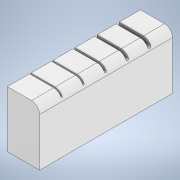
# Autodesk Inventor part: Nut0
Saved by Autodesk Inventor 2021 (Build 250183000, 183)
## iProperties
Created: 2021-02-08
Part Number: Nut0
Material: LCP Plastic
Document SubType Name: Modeling
Designer: Ryan
Density: 1.626 g/cm^3
Appearance: Smooth - White
Author: Ryan
Autodesk Inventor part; units mm, degrees
ref_plane "YZ Plane" through (0, 0, 0) normal (1, 0, 0) x (0, 1, 0)
ref_plane "XZ Plane" through (0, 0, 0) normal (0, 1, 0) x (-1, 0, 0)
ref_plane "XY Plane" through (0, 0, 0) normal (0, 0, 1) x (1, 0, 0)
sketch "Sketch1" plane through (0, 0, 0) normal (0, 1, 0) x (-1, 0, 0)
  line L0 (6.35, 26.2509) -> (-6.35, 26.2509)
  line L1 (-6.35, 26.2509) -> (-6.35, -26.2509)
  line L2 (-6.35, -26.2509) -> (6.35, -26.2509)
  line L3 (6.35, -26.2509) -> (6.35, 26.2509)
  point P0 (0, 0)
  dimension "d0" = 6.35
  dimension "d1" = 12.7
  dimension "d2" = 52.5018
  dimension "d3" = 26.2509
  constraints: 8 end point, 2 parallel, 1 horizontal, 1 perpendicular
  measures "d0" distance from line of point (0, 0) L3
  measures "d1" distance of L0.start L0.end
  measures "d2" distance of L0.end L1.end
  measures "d3" distance from line of L0 point (0, 0)
extrude "Extrusion1" add sketch "Sketch1" along normal blind 22.225
fillet "Fillet1" radius 3.175 1 edges at (6.35, 22.225, 0)
sketch "Sketch2" plane through (-6.35, 0, -26.2509) normal (-1, 0, 0) x (0, 0, 1)
  line L0 (52.5018, 19.05) -> (0, 19.05) projected
  line L1 (0, 0) -> (0, 22.225) projected
  line L2 (52.5018, 0) -> (52.5018, 22.225) projected
  line L3 (8.3439, 22.225) -> (9.6139, 22.225)
  line L4 (9.6139, 22.225) -> (9.6139, 20.447)
  line L5 (9.6139, 20.447) -> (8.3439, 20.447)
  line L6 (8.3439, 20.447) -> (8.3439, 22.225)
  line L7 (17.1069, 22.225) -> (18.1229, 22.225)
  line L8 (18.1229, 22.225) -> (18.1229, 20.447)
  line L9 (18.1229, 20.447) -> (17.1069, 20.447)
  line L10 (17.1069, 20.447) -> (17.1069, 22.225)
  line L11 (25.8699, 22.225) -> (26.6319, 22.225)
  line L12 (26.6319, 22.225) -> (26.6319, 20.447)
  line L13 (26.6319, 20.447) -> (25.8699, 20.447)
  line L14 (25.8699, 20.447) -> (25.8699, 22.225)
  line L15 (34.6075, 22.225) -> (35.1663, 22.225)
  line L16 (35.1663, 22.225) -> (35.1663, 20.447)
  line L17 (35.1663, 20.447) -> (34.6075, 20.447)
  line L18 (34.6075, 20.447) -> (34.6075, 22.225)
  line L19 (43.2689, 22.225) -> (43.7769, 22.225)
  line L20 (43.7769, 22.225) -> (43.7769, 20.447)
  line L21 (43.7769, 20.447) -> (43.2689, 20.447)
  line L22 (43.2689, 20.447) -> (43.2689, 22.225)
  line L23 (8.9789, 20.447) -> (17.6149, 20.447) construction
  line L24 (17.6149, 20.447) -> (26.2509, 20.447) construction
  line L25 (26.2509, 20.447) -> (34.8869, 20.447) construction
  line L26 (34.8869, 20.447) -> (43.5229, 20.447) construction
  arc A0 (8.3439, 20.447) -> (9.6139, 20.447) centre (8.9789, 20.447) ccw
  arc A1 (17.1069, 20.447) -> (18.1229, 20.447) centre (17.6149, 20.447) ccw
  arc A2 (25.8699, 20.447) -> (26.6319, 20.447) centre (26.2509, 20.447) ccw
  arc A3 (34.6075, 20.447) -> (35.1663, 20.447) centre (34.8869, 20.447) ccw
  arc A4 (43.2689, 20.447) -> (43.7769, 20.447) centre (43.5229, 20.447) ccw
  line L27 (34.6075, 22.225) -> (35.1663, 22.225)
  line L28 (43.2689, 22.225) -> (43.7769, 22.225)
  line L29 (25.8699, 22.225) -> (26.6319, 22.225)
  line L30 (8.3439, 22.225) -> (9.6139, 22.225)
  line L31 (17.1069, 22.225) -> (18.1229, 22.225)
  line L32 (0, 22.225) -> (52.5018, 22.225) projected
  line L33 (8.9789, 20.447) -> (0, 20.447) construction
  line L34 (43.5229, 20.447) -> (52.5018, 20.447) construction
  point P0 (26.2509, 0)
  dimension "d20" = 1.27
  dimension "d21" = 1.016
  dimension "d22" = 0.762
  dimension "d23" = 0.508
  dimension "d24" = 0.5588
  dimension "d25" = 1.778
  dimension "d26" = 8.636
  constraints: 62 end point, 20 point on line, 10 parallel, 10 point on circle, 6 perpendicular, 5 centre point, 5 coincident, 5 horizontal, 5 midpoint, 4 collinear
  measures "d20" distance of L4.end L5.end
  measures "d21" distance of L8.end L10.start
  measures "d22" distance of L12.end L14.start
  measures "d23" distance of L20.end L22.start
  measures "d24" distance of L16.end L18.start
  measures "d25" distance of L5.end L3.start
  measures "d26" distance of L23.start L24.start
extrude "Extrusion4" cut sketch "Sketch2" against normal blind 25.4 contours L20 L21 L22 L19 | L3 L4 L5 L6 | A4 L21 | L5 A0 | L16 L17 L18 L15 | L7 L8 L9 L10 | A3 L17 | L9 A1 | L12 L13 L14 L11 | A2 L13
equation "\"d0\" = 0.5 * d1"
equation "\"d3\" = 0.5 * d2"
body "Solid1"
